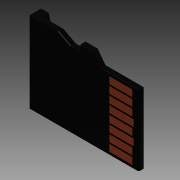
# Autodesk Inventor part: MicroSD
Saved by Autodesk Inventor 2015 (Build 190159000, 159)
## iProperties
Created: 2012-09-09
Part Number: MicroSD
Material: Generic
Document SubType Name: Modeling
Designer: Michael
Density: 1 g/cm^3
Appearance: Default
Mass: 0.135831 g
Surface Area: 3.72268 cm^2
Volume: 0.135831 cm^3
Author: Michael
Autodesk Inventor part; units mm, degrees
ref_plane "YZ Plane" through (0, 0, 0) normal (1, 0, 0) x (0, 1, 0)
ref_plane "XZ Plane" through (0, 0, 0) normal (0, 1, 0) x (-1, 0, 0)
ref_plane "XY Plane" through (0, 0, 0) normal (0, 0, 1) x (1, 0, 0)
sketch "Sketch1" plane through (0, 0, 0) normal (0, 1, 0) x (-1, 0, 0)
  line L0 (-7.53, 4.16) -> (-7.53, -5.59)
  line L1 (-7.53, -5.59) -> (7.53, -5.59)
  line L2 (7.53, -5.59) -> (7.53, 5.59)
  line L3 (7.53, 5.59) -> (-7.53, -5.59) construction
  line L4 (-7.53, 5.59) -> (7.53, -5.59) construction
  line L5 (-7.53, 5.59) -> (-2.34, 5.59) construction
  line L6 (-7.53, -5.59) -> (-7.53, 4.16) construction
  line L7 (-7.53, 4.16) -> (-2.2416, 4.16)
  line L8 (-2.34, 5.59) -> (0.48, 5.59) construction
  line L9 (0.48, 5.59) -> (-1.18, 5.59) construction
  line L10 (-2.2416, 4.16) -> (-1.18, 5.59)
  line L11 (0.48, -5.59) -> (0.48, 4.7) construction
  line L12 (0.48, 5.59) -> (0.48, 4.7)
  line L13 (0.48, 4.7) -> (1.85, 4.7)
  line L14 (1.85, 4.7) -> (3.55, 4.7) construction
  line L15 (1.85, 4.7) -> (3.55, 5.59)
  line L16 (7.53, 5.59) -> (3.55, 5.59)
  line L17 (0.48, 5.59) -> (-1.18, 5.59)
  point P0 (0, 0)
  dimension "d0" = 15.06
  dimension "d1" = 11.18
  dimension "d2" = 5.19
  dimension "d3" = 9.75
  dimension "d4" = 2.82
  dimension "d5" = 1.66
  dimension "d6" = 10.29
  dimension "d7" = 1.37
  dimension "d8" = 1.7
  constraints: 36 end point, 6 perpendicular, 5 parallel, 2 horizontal, 2 midpoint, 2 point on line, 1 collinear
  measures "d0" distance of L1.end L0.end
  measures "d1" distance of L0.end L4.start
  measures "d2" distance of L4.start L5.end
  measures "d3" distance of L0.start L0.end
  measures "d4" distance of L5.end L8.end
  measures "d5" distance of L9.end L8.end
  measures "d6" distance of L11.start L11.end
  measures "d7" distance of L11.end L13.end
  measures "d8" distance of L13.end L14.end
extrude "Extrusion1" add sketch "Sketch1" along normal blind 0.75
sketch "Sketch2" plane through (0, 0.75, 0) normal (0, 1, 0) x (1, 0, 0)
  line L0 (-7.53, 5.59) -> (-7.53, -5.59) projected
  line L1 (-7.53, -5.59) -> (-3.55, -5.59) projected
  line L2 (7.53, 5.59) -> (-7.53, 5.59) projected
  line L3 (-7.53, 5.59) -> (-6.33, 5.59) construction
  line L4 (-7.53, -5.59) -> (-6.33, -5.59) construction
  line L5 (-7.53, 0) -> (-5.42, 0) construction
  arc A0 (-6.33, -5.59) -> (-6.33, 5.59) centre (-23.0443, 0) ccw
  point P0 (0, 0)
  dimension "d11" = 1.2
  dimension "d12" = 2.11
  constraints: 6 end point, 3 point on circle, 2 point on line, 1 centre point, 1 midpoint, 1 parallel
  measures "d11" distance of L0.start L3.end
  measures "d12" distance of L5.start L5.end
extrude "Extrusion2" add sketch "Sketch2" along normal blind 0.9
fillet "Fillet1" radius 0.3 1 edges at (-5.42, 1.65, 0)
fillet "Fillet2" radius 0.1 29 edges at (-5.42, 0.75, 0) (-4.94, 0.75, 5.59) (-2.7, 0.75, 5.145) (-1.165, 0.75, 4.7) (-0.48, 0.75, 5.145) (0.35, 0.75, 5.59) (1.7108, 0.75, 4.875) (4.8858, 0.75, 4.16) (7.53, 0.75, -0.715) (0.6, 0.75, -5.59) (4.8858, 0, 4.16) (1.7108, 0, 4.875) (0.35, 0, 5.59) (-2.7, 0, 5.145) (-1.165, 0, 4.7) (-5.54, 0, 5.59) (-7.53, 0.825, 5.59) (-7.53, 0, 0) (-7.53, 1.65, 0) (-7.53, 0.825, -5.59) (0, 0, -5.59) (7.53, 0.375, 4.16) (7.53, 0.375, -5.59) (-6.33, 1.05, 5.59) (-7.0883, 1.65, 5.59) (-6.4229, 1.5624, 5.59) (-7.0883, 1.65, -5.59) (-6.33, 1.05, -5.59) (-6.4229, 1.5624, -5.59)
sketch "Sketch3" plane through (0, 0, 0) normal (0, -1, 0) x (1, 0, 0)
  line L0 (7.53, -5.49) -> (-7.43, -5.49) projected
  line L1 (7.43, 4.06) -> (7.43, -5.49) projected
  line L2 (2.1913, 4.06) -> (7.53, 4.06) projected
  line L3 (7.43, -0.715) -> (3.38, -0.715) construction
  line L4 (3.38, 4.06) -> (3.38, -5.49)
  point P0 (0, 0)
  dimension "d17" = 4.05
  constraints: 4 end point, 2 point on line, 1 midpoint, 1 parallel, 1 perpendicular
  measures "d17" distance of L3.start L3.end
extrude "Extrusion3" cut sketch "Sketch3" against normal blind 0.02
sketch "Sketch4" plane through (7.43, 0, -5.49) normal (-1, 0, 0) x (0, 0, 1)
  line L0 (9.55, 0) -> (0, 0) projected
  line L1 (9.55, 0) -> (9.55, 0.02) projected
  line L2 (9.55, 0.02) -> (0, 0.02) projected
  line L3 (0, 0) -> (0, 0.02) projected
  point P0 (5.49, 0)
extrude "Extrusion4" cut sketch "Sketch4" against normal blind 1
sketch "Sketch5" plane through (0, 0.02, 0) normal (0, -1, 0) x (1, 0, 0)
  line L0 (3.38, 4.06) -> (7.53, 4.06) projected
  line L1 (3.38, -5.49) -> (3.38, 4.06) projected
  line L2 (7.53, -5.49) -> (3.38, -5.49) projected
  line L3 (6.64, -5.19) -> (3.48, -5.19)
  line L4 (3.48, -5.19) -> (3.48, -4.29)
  line L5 (3.48, -4.29) -> (6.64, -4.29)
  line L6 (6.64, -4.29) -> (6.64, -5.19)
  line L7 (6.64, -5.19) -> (3.48, -4.29) construction
  line L8 (3.48, -5.19) -> (6.64, -4.29) construction
  line L9 (6.64, -4.04) -> (3.48, -4.04)
  line L10 (3.48, -4.04) -> (3.48, -3.14)
  line L11 (3.48, -3.14) -> (6.64, -3.14)
  line L12 (6.64, -3.14) -> (6.64, -4.04)
  line L13 (6.64, -4.04) -> (3.48, -3.14) construction
  line L14 (3.48, -4.04) -> (6.64, -3.14) construction
  line L15 (6.64, -1.74) -> (3.48, -1.74)
  line L16 (3.48, -1.74) -> (3.48, -0.84)
  line L17 (3.48, -0.84) -> (6.64, -0.84)
  line L18 (6.64, -0.84) -> (6.64, -1.74)
  line L19 (6.64, -1.74) -> (3.48, -0.84) construction
  line L20 (3.48, -1.74) -> (6.64, -0.84) construction
  line L21 (6.64, 0.56) -> (3.48, 0.56)
  line L22 (3.48, 0.56) -> (3.48, 1.46)
  line L23 (3.48, 1.46) -> (6.64, 1.46)
  line L24 (6.64, 1.46) -> (6.64, 0.56)
  line L25 (6.64, 0.56) -> (3.48, 1.46) construction
  line L26 (3.48, 0.56) -> (6.64, 1.46) construction
  line L27 (6.64, 1.71) -> (3.48, 1.71)
  line L28 (3.48, 1.71) -> (3.48, 2.61)
  line L29 (3.48, 2.61) -> (6.64, 2.61)
  line L30 (6.64, 2.61) -> (6.64, 1.71)
  line L31 (6.64, 1.71) -> (3.48, 2.61) construction
  line L32 (3.48, 1.71) -> (6.64, 2.61) construction
  line L33 (6.64, 2.86) -> (3.48, 2.86)
  line L34 (3.48, 2.86) -> (3.48, 3.76)
  line L35 (3.48, 3.76) -> (6.64, 3.76)
  line L36 (6.64, 3.76) -> (6.64, 2.86)
  line L37 (6.64, 2.86) -> (3.48, 3.76) construction
  line L38 (3.48, 2.86) -> (6.64, 3.76) construction
  line L39 (3.48, -2.89) -> (6.81, -2.89)
  line L40 (6.81, -2.89) -> (6.81, -1.99)
  line L41 (6.81, -1.99) -> (3.48, -1.99)
  line L42 (3.48, -1.99) -> (3.48, -2.89)
  line L43 (3.48, -2.89) -> (6.81, -1.99) construction
  line L44 (6.81, -2.89) -> (3.48, -1.99) construction
  line L45 (3.48, -0.59) -> (6.81, -0.59)
  line L46 (6.81, -0.59) -> (6.81, 0.31)
  line L47 (6.81, 0.31) -> (3.48, 0.31)
  line L48 (3.48, 0.31) -> (3.48, -0.59)
  line L49 (3.48, -0.59) -> (6.81, 0.31) construction
  line L50 (6.81, -0.59) -> (3.48, 0.31) construction
  point P0 (7.49, 4.06)
  point P1 (7.49, -5.49)
  point P2 (0, 0)
  point P3 (5.06, -4.74)
  point P4 (5.06, -3.59)
  point P5 (5.06, -1.29)
  point P6 (5.06, 1.01)
  point P7 (5.06, 2.16)
  point P8 (5.06, 3.31)
  point P9 (5.145, -2.44)
  point P10 (5.145, -0.14)
  dimension "d22" = 3.16
  dimension "d23" = 0.9
  dimension "d24" = 0.3
  dimension "d25" = 0.1
  dimension "d26" = 3.16
  dimension "d27" = 0.9
  dimension "d28" = 3.16
  dimension "d29" = 0.9
  dimension "d30" = 3.16
  dimension "d31" = 0.9
  dimension "d32" = 3.16
  dimension "d33" = 0.9
  dimension "d34" = 3.16
  dimension "d35" = 0.9
  dimension "d36" = 0.25
  dimension "d37" = 0.25
  dimension "d39" = 0.25
  dimension "d41" = 3.33
  dimension "d42" = 0.9
  dimension "d43" = 0.1
  dimension "d44" = 0.25
  dimension "d45" = 0.25
  dimension "d46" = 3.33
  dimension "d47" = 0.9
  dimension "d48" = 0.25
  dimension "d49" = 0.25
  dimension "d50" = 0.3
  constraints: 96 end point, 16 midpoint, 16 parallel, 8 horizontal, 8 perpendicular
  measures "d22" distance of L4.end L5.end
  measures "d23" distance of L3.end L4.end
  measures "d24" distance between parallel lines of L2 L3
  measures "d25" distance between parallel lines of L1 L4
  measures "d26" distance of L10.end L11.end
  measures "d27" distance of L9.end L10.end
  measures "d28" distance of L16.end L17.end
  measures "d29" distance of L15.end L16.end
  measures "d30" distance of L22.end L23.end
  measures "d31" distance of L21.end L22.end
  measures "d32" distance of L28.end L29.end
  measures "d33" distance of L27.end L28.end
  measures "d34" distance of L34.end L35.end
  measures "d35" distance of L33.end L34.end
  measures "d36" distance between parallel lines of L5 L9
  measures "d37" distance between parallel lines of L27 L23
  measures "d39" distance between parallel lines of L33 L29
  measures "d41" distance of L41.end L40.end
  measures "d42" distance of L40.end L39.end
  measures "d43" distance between parallel lines of L1 L42
  measures "d44" distance between parallel lines of L41 L15
  measures "d45" distance between parallel lines of L11 L39
  measures "d46" distance of L48.start L46.end
  measures "d47" distance of L46.end L45.end
  measures "d48" distance between parallel lines of L45 L17
  measures "d49" distance between parallel lines of L21 L47
  measures "d50" distance between parallel lines of L35 L0
extrude "Extrusion5" add sketch "Sketch5" along normal blind 0.02
chamfer "Chamfer1" distance 0.2 angle 45 1 edges at (7.53, 0.02, -0.715)
sketch "Sketch6" plane through (3.38, 0, -5.49) normal (0, 0, 1) x (1, 0, 0)
  line L0 (4.15, 0) -> (0, 0) projected
  line L1 (4.15, 0.22) -> (4.15, 0) projected
  line L2 (4.15, 0.22) -> (3.95, 0.02) projected
  line L3 (3.95, 0.02) -> (3.93, 0)
  point P0 (-3.38, 0)
  constraints: 2 end point, 1 collinear, 1 point on line
extrude "Extrusion6" cut sketch "Sketch6" against normal blind 1
sketch "Sketch7" plane through (7.53, 0, 4.06) normal (0, 0, -1) x (-1, 0, 0)
  line L0 (4.15, 0) -> (0, 0) projected
  line L1 (0, 0.22) -> (0.2, 0.02) projected
  line L2 (0, 0) -> (0, 0.22) projected
  line L3 (0.2, 0.02) -> (0.22, 0)
  point P0 (7.53, 0)
  constraints: 2 end point, 1 collinear, 1 point on line
extrude "Extrusion7" cut sketch "Sketch7" against normal blind 1
body "Solid1"
